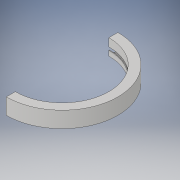
# Autodesk Inventor part: OuterShell_Top_Quarter
Saved by Autodesk Inventor 2017 (Build 210142000, 142)
## iProperties
Created: 2017-01-20
Part Number: OuterShell_Top_Quarter
Material: Generic
Document SubType Name: Modeling
Designer: David Kopala
Density: 1 g/cm^3
Appearance: Default
IDia: 10.500 in
Wall: 0.063 in
Space: 0.063 in
SpWall: 0.125 in
IBDia: 10.989 in
BevOutInDia: 11.323 in
BevOutOutDia: 11.721 in
BevDriverDia: 0.936 in
d1_1: 0.250 in
AxelDia: 0.250 in
Author: David Kopala
Autodesk Inventor part; units mm, degrees
ref_plane "YZ Plane" through (0, 0, 0) normal (1, 0, 0) x (0, 1, 0)
ref_plane "XZ Plane" through (0, 0, 0) normal (0, 1, 0) x (-1, 0, 0)
ref_plane "XY Plane" through (0, 0, 0) normal (0, 0, 1) x (1, 0, 0)
sketch "Sketch1" plane through (0, 0, 0) normal (1, 0, 0) x (0, 1, 0)
  line L0 (0, 0) -> (73.993, 0)
  line L1 (0, 130.0359) -> (44.4227, 130.0359)
  line L2 (0, 130.0359) -> (0, 155.2107)
  line L3 (0, 155.2107) -> (44.4227, 155.2107)
  line L4 (44.4227, 155.2107) -> (44.4227, 130.0359)
  line L5 (42.8352, 153.6232) -> (1.5875, 153.6232)
  line L6 (1.5875, 153.6232) -> (1.5875, 131.6234)
  line L7 (1.5875, 131.6234) -> (42.8352, 131.6234)
  line L8 (42.8352, 131.6234) -> (42.8352, 153.6232)
  line L9 (18.2426, 143.1015) -> (18.2426, 119.3292)
  line L10 (14.2738, 131.6234) -> (14.2738, 130.0359)
  line L11 (22.2113, 131.6234) -> (22.2113, 130.0359)
  dimension "d1" = 25.1748
  dimension "d2" = 130.0359
  dimension "d3" = 44.4227
  dimension "d4" = 0
  dimension "d5" = 1.5875
  dimension "d6" = 1.5875
  dimension "d7" = 1.5875
  dimension "d8" = 1.5875
  dimension "d9" = 18.2426
  dimension "d10" = 7.9375
  dimension "d11" = 3.9688
  constraints: 24 end point, 4 horizontal, 3 perpendicular, 2 midpoint, 2 parallel, 2 point on line, 2 vertical
  measures "d1" distance of L1.start L2.end
  measures "d2" distance between parallel lines of L0 L1
  measures "d3" distance of L2.end L3.end
  measures "d4" horizontal distance of L1.end L3.end
  measures "d5" distance from line of L3 L5.start
  measures "d6" distance from line of L4 L5.start
  measures "d7" distance from line of L2 L6.end
  measures "d8" distance from line of L6.end L1
  measures "d9" distance between parallel lines of L2 L9
  measures "d10" distance between parallel lines of L10 L11
  measures "d11" distance between parallel lines of L10 L9
revolve "Revolution1" add sketch "Sketch1" angle 180 about axis through (0, 0, 0) along (0, 1, 0) contours L2 L3 L4 L1 L11 L7 L8 L5 L6 L10
equation "\"d2\" = 0.5 * IBDia - 3 * SpWall"
equation "\"d3\" = Wall + 4 * SpWall + BevDriverDia + d1_1"
equation "\"d5\" = Wall"
equation "\"d6\" = Wall"
equation "\"d7\" = Wall"
equation "\"d8\" = Wall"
equation "\"d9\" = 2 * SpWall + 0.5 * BevDriverDia"
equation "\"d10\" = AxelDia + Space"
equation "\"d11\" = 0.5 * Space + 0.5 * AxelDia"
equation "\"IDia\" = 266.7"
equation "\"Wall\" = 1.5875"
equation "\"Space\" = 1.5875"
equation "\"SpWall\" = 3.175"
equation "\"AxelDia\" = 6.35"
equation "\"IBDia\" = 279.121792"
equation "\"BevDriverDia\" = 23.785175"
equation "\"d1_1\" = 6.35"
body "Solid1"
